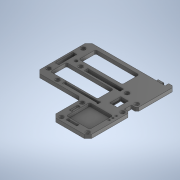
# Autodesk Inventor part: Cockpit_side_frame
Saved by Autodesk Inventor 2020.4 (Build 244396000, 396)
## iProperties
Created: 2022-01-27
Part Number: Cockpit_side_frame
Material: アセタール樹脂、黒
Document SubType Name: Modeling
Designer: Masato Kubotera
Density: 1.425 g/cm^3
Appearance: 滑らか - 黒
Mass: 53.6931 g
Surface Area: 240.102 cm^2
Volume: 37.6794 cm^3
Description: POM T5
Author: Masato Kubotera
Autodesk Inventor part; units mm, degrees
ref_plane "YZ Plane" through (0, 0, 0) normal (1, 0, 0) x (0, 1, 0)
ref_plane "XZ Plane" through (0, 0, 0) normal (0, 1, 0) x (-1, 0, 0)
ref_plane "XY Plane" through (0, 0, 0) normal (0, 0, 1) x (1, 0, 0)
derived "Trunk_basis.ipt"
sketch "スケッチ1" plane through (0, 0, 0) normal (0, 1, 0) x (-1, 0, 0)
  line L0 (0, 22) -> (0, -142.9) construction
  circle A0 centre (5, 0) radius 10.5 construction
  line L1 (-7, 16) -> (36, 16) construction
  line L2 (36, 16) -> (36, -16) construction
  line L3 (36, -16) -> (-7, -16) construction
  line L4 (-7, -16) -> (-7, 16) construction
  line L5 (-7, 16) -> (36, -16) construction
  line L6 (36, 16) -> (-7, -16) construction
  line L7 (33, 13.5) -> (6, 13.5) construction
  line L8 (6, 13.5) -> (6, -13.5) construction
  line L9 (6, -13.5) -> (33, -13.5) construction
  line L10 (33, -13.5) -> (33, 13.5) construction
  line L11 (33, 13.5) -> (6, -13.5) construction
  line L12 (6, 13.5) -> (33, -13.5) construction
  line L13 (-7, 0) -> (36, 0) construction
  arc A1 (5, 16) -> (-7, 10.583) centre (5, 0) ccw construction
  line L14 (34.5651, -16.05) -> (5, -16.05)
  line L15 (5, 16.05) -> (34.5651, 16.05)
  line L16 (36.05, 14.5651) -> (36.05, -14.5651)
  line L17 (36.05, -16.05) -> (-7.05, 16.05) construction
  line L18 (-7.05, -16.05) -> (36.05, 16.05) construction
  arc A2 (5, 16.05) -> (-6.5314, 11.1638) centre (5, 0) ccw
  arc A3 (-6.5314, 11.1638) -> (-7.05, 9.8372) centre (-6.0721, 10.2196) ccw
  arc A4 (36.05, 14.5651) -> (34.5651, 16.05) centre (35.3075, 15.3075) ccw
  circle A5 centre (6, 13.5) radius 1.35
  line L19 (19.5, 13.5) -> (19.5, -13.5) construction
  circle A6 centre (33, 13.5) radius 1.35
  line L20 (-15, 22) -> (-20, 17)
  line L21 (-20, 17) -> (-20, -19)
  line L22 (-20, -19) -> (-28.5, -27.5)
  line L23 (-28.5, -27.5) -> (-28.5, -103)
  line L24 (57.5, -22.5) -> (57.5, 17)
  line L25 (57.5, 17) -> (52.5, 22)
  line L26 (52.5, 22) -> (-15, 22)
  line L27 (-35.5597, -116.5529) -> (-28.5, -142.9)
  line L28 (-16, -139) -> (-16, -94) construction
  line L29 (-7.5, -140.4849) -> (-7.5, -142.9)
  line L30 (-7.5, -142.9) -> (7.5, -142.9)
  line L31 (7.5, -140.4849) -> (7.5, -142.9)
  arc A7 (-7.5, -140.4849) -> (-8.9849, -139) centre (-8.2425, -139.7425) ccw
  line L32 (-17.5, -138.9955) -> (-17.5, -133) construction
  line L33 (-19, -133) -> (-16, -133) construction
  line L34 (-19, -133) -> (-19, -139) construction
  line L35 (-16, -133) -> (-16, -139) construction
  line L36 (-15, 22) -> (-10, 22) construction
  line L37 (-10, 22) -> (-10, -22) construction
  line L38 (-10, -22) -> (-15, -22) construction
  line L39 (-15, -22) -> (-15, 22) construction
  line L40 (-15, 22) -> (-10, -22) construction
  line L41 (-10, 22) -> (-15, -22) construction
  line L42 (-12.5, 22) -> (-12.5, -22) construction
  line L43 (-10, 0) -> (-15, 0) construction
  circle A8 centre (-12.5, 17.75) radius 1.6
  line L44 (-15, 10) -> (-12.5, 10) construction
  line L45 (-12.5, 10) -> (-12.5, -10) construction
  line L46 (-12.5, -10) -> (-15, -10) construction
  line L47 (-15, -10) -> (-15, 10) construction
  line L48 (-15, 10) -> (-12.5, -10) construction
  line L49 (-12.5, 10) -> (-15, -10) construction
  line L50 (-12.45, 10.05) -> (-15.05, 10.05)
  line L51 (-15.05, 7.95) -> (-15.05, -7.95)
  line L52 (-15.05, -10.05) -> (-12.45, -10.05)
  line L53 (-12.45, -7.95) -> (-12.45, 7.95)
  line L54 (-12.45, 10.05) -> (-15.05, -10.05) construction
  line L55 (-15.05, 10.05) -> (-12.45, -10.05) construction
  arc A9 (-15.05, 10.05) -> (-15.05, 7.95) centre (-15.05, 9) ccw
  line L56 (-13.75, 10) -> (-13.75, -10) construction
  arc A10 (-12.45, 7.95) -> (-12.45, 10.05) centre (-12.45, 9) ccw
  circle A11 centre (-12.5, -17.75) radius 1.6
  arc A12 (-15.05, -7.95) -> (-15.05, -10.05) centre (-15.05, -9) ccw
  arc A13 (-12.45, -10.05) -> (-12.45, -7.95) centre (-12.45, -9) ccw
  line L57 (36, 14.4) -> (44.5, 14.4) construction
  line L58 (44.5, 14.4) -> (44.5, -14.4) construction
  line L59 (36, -14.4) -> (44.5, -14.4) construction
  line L60 (49.95, 7.95) -> (49.95, -7.95)
  line L61 (52.5, 0) -> (47.5, 0) construction
  line L62 (47.5, 22) -> (52.5, 22) construction
  line L63 (52.55, -7.95) -> (52.55, 7.95)
  line L64 (51.25, 10) -> (51.25, -10) construction
  line L65 (52.5, 10) -> (50, -10) construction
  line L66 (52.5, -10) -> (50, -10) construction
  line L67 (52.5, 10) -> (52.5, -10) construction
  line L68 (50, 10) -> (52.5, -10) construction
  line L69 (49.95, -10.05) -> (52.55, -10.05)
  line L70 (49.95, 10.05) -> (52.55, -10.05) construction
  line L71 (52.55, 10.05) -> (49.95, -10.05) construction
  line L72 (52.5, -22) -> (47.5, -22) construction
  line L73 (47.5, 22) -> (52.5, -22) construction
  line L74 (52.5, 22) -> (52.5, -22) construction
  line L75 (52.5, 22) -> (47.5, -22) construction
  line L76 (50, 22) -> (50, -22) construction
  line L77 (47.5, -22) -> (47.5, 22) construction
  circle A14 centre (50, -17.75) radius 1.6
  arc A15 (52.55, -10.05) -> (52.55, -7.95) centre (52.55, -9) ccw
  line L78 (50, -10) -> (50, 10) construction
  arc A16 (49.95, -7.95) -> (49.95, -10.05) centre (49.95, -9) ccw
  arc A17 (49.95, 10.05) -> (49.95, 7.95) centre (49.95, 9) ccw
  arc A18 (52.55, 7.95) -> (52.55, 10.05) centre (52.55, 9) ccw
  line L79 (50, 10) -> (52.5, 10) construction
  line L80 (52.55, 10.05) -> (49.95, 10.05)
  circle A19 centre (50, 17.75) radius 1.6
  circle A20 centre (5, 0) radius 16 construction
  arc A21 (-6.5314, -11.1638) -> (5, -16.05) centre (5, 0) ccw
  arc A22 (-7.05, -9.8372) -> (-6.5314, -11.1638) centre (-6.0721, -10.2196) ccw
  arc A23 (34.5651, -16.05) -> (36.05, -14.5651) centre (35.3075, -15.3075) ccw
  line L81 (-7.05, -9.8372) -> (-7.05, 9.8372)
  line L82 (17.5, -138.9955) -> (17.5, -133) construction
  line L83 (19, -133) -> (19, -139) construction
  line L84 (16, -133) -> (16, -139) construction
  line L85 (19, -133) -> (16, -133) construction
  circle A24 centre (6, -13.5) radius 1.35
  circle A25 centre (33, -13.5) radius 1.35
  line L86 (-25.5, -142.9) -> (-7.5, -142.9) construction
  line L87 (25.5, -142.9) -> (7.5, -142.9) construction
  line L88 (-23.5, -22.5) -> (57.5, -22.5) construction
  line L89 (57.5, -22.5) -> (57.5, -103)
  circle A26 centre (-13.5, -55) radius 1.75
  line L90 (-16.5, -59) -> (45.5, -59)
  line L91 (47.5, -61) -> (47.5, -88)
  line L92 (45.5, -90) -> (-16.5, -90)
  line L93 (-18.5, -88) -> (-18.5, -61)
  line L94 (-18.5, -59) -> (47.5, -90) construction
  line L95 (47.5, -59) -> (-18.5, -90) construction
  line L96 (-16.5, -27.5) -> (45.5, -27.5)
  line L97 (47.5, -29.5) -> (47.5, -49)
  line L98 (45.5, -51) -> (-16.5, -51)
  line L99 (-18.5, -49) -> (-18.5, -29.5)
  line L100 (-18.5, -27.5) -> (47.5, -51) construction
  line L101 (47.5, -27.5) -> (-18.5, -51) construction
  line L102 (-23.5, -108) -> (-28.5, -103)
  circle A27 centre (-20.5415, -102) radius 1.6
  line L103 (-25.7227, -96) -> (25.7227, -96)
  line L104 (25.7227, -96) -> (34.9603, -112)
  line L105 (35.5597, -116.5529) -> (28.5, -142.9)
  line L106 (-25.7227, -96) -> (-34.9603, -112)
  line L107 (57.5, -103) -> (52.5, -108)
  arc A28 (-16.5, -27.5) -> (-18.5, -29.5) centre (-16.5, -29.5) ccw
  arc A29 (-18.5, -49) -> (-16.5, -51) centre (-16.5, -49) ccw
  arc A30 (45.5, -51) -> (47.5, -49) centre (45.5, -49) ccw
  arc A31 (47.5, -29.5) -> (45.5, -27.5) centre (45.5, -29.5) ccw
  arc A32 (-16.5, -59) -> (-18.5, -61) centre (-16.5, -61) ccw
  arc A33 (-18.5, -88) -> (-16.5, -90) centre (-16.5, -88) ccw
  arc A34 (45.5, -90) -> (47.5, -88) centre (45.5, -88) ccw
  arc A35 (47.5, -61) -> (45.5, -59) centre (45.5, -61) ccw
  line L108 (-23.5, -108) -> (52.5, -108)
  line L109 (-25.5, -139) -> (-25.5, -142.9)
  line L110 (-25.5, -142.9) -> (-28.5, -142.9)
  line L111 (-17.9813, -99.3843) -> (-16.9961, -101.0907)
  line L112 (-16.9961, -102.9093) -> (-17.9813, -104.6157)
  line L113 (-19.5563, -105.525) -> (-21.5266, -105.525)
  line L114 (-23.1016, -104.6157) -> (-24.0868, -102.9093)
  line L115 (-24.0868, -101.0907) -> (-23.1016, -99.3843)
  line L116 (-21.5266, -98.475) -> (-19.5563, -98.475)
  line L117 (-16, -94) -> (16, -94) construction
  arc A36 (-24.0868, -101.0907) -> (-24.0868, -102.9093) centre (-23.5618, -102) ccw
  arc A37 (-23.1016, -104.6157) -> (-21.5266, -105.525) centre (-22.0516, -104.6157) ccw
  arc A38 (-19.5563, -105.525) -> (-17.9813, -104.6157) centre (-19.0313, -104.6157) ccw
  arc A39 (-16.9961, -102.9093) -> (-16.9961, -101.0907) centre (-17.5211, -102) ccw
  arc A40 (-17.9813, -99.3843) -> (-19.5563, -98.475) centre (-19.0313, -99.3843) ccw
  arc A41 (-21.5266, -98.475) -> (-23.1016, -99.3843) centre (-22.0516, -99.3843) ccw
  line L118 (16, -139) -> (16, -94) construction
  line L119 (16, -94) -> (-16, -94) construction
  line L120 (-25.5, -139) -> (-8.9849, -139)
  line L121 (25.5, -142.9) -> (28.5, -142.9)
  arc A42 (8.9849, -139) -> (7.5, -140.4849) centre (8.2425, -139.7425) ccw
  circle A43 centre (29.7641, -115) radius 1.25
  line L122 (33.4891, -124.2803) -> (21.898, -121.1745) construction
  line L123 (29.7641, -115) -> (25.623, -130.4548) construction
  circle A44 centre (29.7641, -115) radius 6 construction
  circle A45 centre (-20.5415, -102) radius 6 construction
  line L124 (1.9319, -109.4824) -> (7.5588, -130.4824)
  line L125 (5.6269, -133) -> (-5.6269, -133)
  line L126 (5.3151, -110.5176) -> (10.942, -131.5176)
  line L127 (12.8739, -133) -> (17.1947, -133)
  line L128 (19.1266, -131.5176) -> (24.7535, -110.5176)
  line L129 (22.8217, -108) -> (7.2469, -108)
  circle A46 centre (25.623, -130.4548) radius 1.25
  circle A47 centre (25.623, -130.4548) radius 6 construction
  line L130 (-1.9319, -109.4824) -> (-7.5588, -130.4824)
  arc A48 (1.9319, -109.4824) -> (-1.9319, -109.4824) centre (0, -110) ccw
  arc A49 (-7.5588, -130.4824) -> (-5.6269, -133) centre (-5.6269, -131) ccw
  arc A50 (5.6269, -133) -> (7.5588, -130.4824) centre (5.6269, -131) ccw
  arc A51 (7.2469, -108) -> (5.3151, -110.5176) centre (7.2469, -110) ccw
  arc A52 (24.7535, -110.5176) -> (22.8217, -108) centre (22.8217, -110) ccw
  arc A53 (17.1947, -133) -> (19.1266, -131.5176) centre (17.1947, -131) ccw
  arc A54 (10.942, -131.5176) -> (12.8739, -133) centre (12.8739, -131) ccw
  arc A55 (-5.3151, -110.5176) -> (-7.2469, -108) centre (-7.2469, -110) ccw
  line L131 (-22.8217, -108) -> (-7.2469, -108)
  line L132 (-5.3151, -110.5176) -> (-10.942, -131.5176)
  arc A56 (-22.8217, -108) -> (-24.7535, -110.5176) centre (-22.8217, -110) ccw
  line L133 (-19.1266, -131.5176) -> (-24.7535, -110.5176)
  arc A57 (-19.1266, -131.5176) -> (-17.1947, -133) centre (-17.1947, -131) ccw
  line L134 (-12.8739, -133) -> (-17.1947, -133)
  arc A58 (-12.8739, -133) -> (-10.942, -131.5176) centre (-12.8739, -131) ccw
  circle A59 centre (-29.7641, -115) radius 1.25
  circle A60 centre (-25.623, -130.4548) radius 1.25
  arc A61 (35.5597, -116.5529) -> (34.9603, -112) centre (29.7641, -115) ccw
  arc A62 (-34.9603, -112) -> (-35.5597, -116.5529) centre (-29.7641, -115) ccw
  arc A63 (-24.0151, -139) -> (-25.5, -140.4849) centre (-24.7575, -139.7425) ccw
  line L135 (25.5, -139) -> (25.5, -142.9)
  arc A64 (25.5, -140.4849) -> (24.0151, -139) centre (24.7575, -139.7425) ccw
  line L136 (25.5, -139) -> (8.9849, -139)
  line L137 (21.5266, -98.475) -> (19.5563, -98.475)
  line L138 (16.9961, -102.9093) -> (17.9813, -104.6157)
  arc A65 (21.5266, -105.525) -> (23.1016, -104.6157) centre (22.0516, -104.6157) ccw
  circle A66 centre (20.5415, -102) radius 1.6
  line L139 (24.0868, -101.0907) -> (23.1016, -99.3843)
  arc A67 (24.0868, -102.9093) -> (24.0868, -101.0907) centre (23.5618, -102) ccw
  line L140 (23.1016, -104.6157) -> (24.0868, -102.9093)
  arc A68 (23.1016, -99.3843) -> (21.5266, -98.475) centre (22.0516, -99.3843) ccw
  line L141 (19.5563, -105.525) -> (21.5266, -105.525)
  arc A69 (19.5563, -98.475) -> (17.9813, -99.3843) centre (19.0313, -99.3843) ccw
  arc A70 (17.9813, -104.6157) -> (19.5563, -105.525) centre (19.0313, -104.6157) ccw
  line L142 (17.9813, -99.3843) -> (16.9961, -101.0907)
  arc A71 (16.9961, -101.0907) -> (16.9961, -102.9093) centre (17.5211, -102) ccw
  line L143 (16, -139) -> (16, -94) construction
  circle A72 centre (20.5415, -102) radius 6 construction
  arc A73 (29.5045, -117.5445) -> (31.2612, -117.0738) centre (30.247, -116.802) ccw construction
  line L144 (31.8379, -116.4971) -> (31.2612, -117.0738) construction
  line L145 (29.5045, -117.5445) -> (28.7167, -117.3334) construction
  arc A74 (27.4307, -116.0474) -> (28.7167, -117.3334) centre (28.4449, -116.3192) ccw construction
  line L146 (27.4307, -116.0474) -> (27.2196, -115.2596) construction
  line L147 (27.6903, -113.5029) -> (28.267, -112.9262) construction
  arc A75 (30.0237, -112.4555) -> (28.267, -112.9262) centre (29.2813, -113.198) ccw construction
  arc A76 (27.6903, -113.5029) -> (27.2196, -115.2596) centre (27.9621, -114.5171) ccw construction
  line L148 (30.0237, -112.4555) -> (30.8116, -112.6666) construction
  arc A77 (31.8379, -116.4971) -> (32.3086, -114.7404) centre (31.5662, -115.4829) ccw construction
  arc A78 (32.0975, -113.9526) -> (30.8116, -112.6666) centre (31.0833, -113.6808) ccw construction
  line L149 (32.0975, -113.9526) -> (32.3086, -114.7404) construction
  line L150 (-20.5415, -102) -> (20.5415, -102) construction
  circle A79 centre (0, -102) radius 1.6
  line L151 (0.4078, -104.525) -> (-0.4078, -104.525)
  arc A80 (-0.4078, -99.475) -> (-1.9828, -100.3843) centre (-0.9328, -100.3843) ccw
  arc A81 (0.4078, -104.525) -> (1.9828, -103.6157) centre (0.9328, -103.6157) ccw
  line L152 (2.3906, -102.9093) -> (1.9828, -103.6157)
  line L153 (-0.4078, -99.475) -> (0.4078, -99.475)
  arc A82 (1.9828, -100.3843) -> (0.4078, -99.475) centre (0.9328, -100.3843) ccw
  line L154 (1.9828, -100.3843) -> (2.3906, -101.0907)
  arc A83 (2.3906, -102.9093) -> (2.3906, -101.0907) centre (1.8656, -102) ccw
  line L155 (-2.3906, -101.0907) -> (-1.9828, -100.3843)
  arc A84 (-2.3906, -101.0907) -> (-2.3906, -102.9093) centre (-1.8656, -102) ccw
  line L156 (-1.9828, -103.6157) -> (-2.3906, -102.9093)
  arc A85 (-1.9828, -103.6157) -> (-0.4078, -104.525) centre (-0.9328, -103.6157) ccw
  circle A86 centre (0, -102) radius 1.25
  point P0 (0, 0)
  point P1 (14.5, 0)
  point P2 (19.5, 0)
  point P3 (-7.05, 10.6019)
  point P4 (19.5, 0)
  point P5 (-12.5, 0)
  point P6 (-13.75, 0)
  point P7 (36.05, 14.4)
  point P8 (36.05, -14.4)
  point P9 (51.25, 0)
  point P10 (50, 0)
  point P11 (14.5, -74.5)
  point P12 (14.5, -39.25)
  point P13 (-18.5063, -98.475)
  point P14 (-16.4711, -102)
  point P15 (-18.5063, -105.525)
  point P16 (-22.5766, -105.525)
  point P17 (-22.5766, -98.475)
  point P18 (-24.6118, -102)
  point P19 (-22.5766, -105.525)
  point P20 (-18.5063, -105.525)
  point P21 (-16.4711, -102)
  point P22 (-18.5063, -98.475)
  point P23 (-22.5766, -98.475)
  point P24 (27.6936, -122.7274)
  point P25 (0, -102.2726)
  point P26 (0, -133)
  point P27 (-7.5, -139)
  point P28 (-22.5766, -98.475)
  point P29 (18.5063, -98.475)
  point P30 (18.5063, -98.475)
  point P31 (22.5766, -105.525)
  point P32 (22.5766, -105.525)
  point P33 (24.6118, -102)
  point P34 (22.5766, -98.475)
  point P35 (22.5766, -98.475)
  point P36 (22.5766, -98.475)
  point P37 (18.5063, -105.525)
  point P38 (16.4711, -102)
  point P39 (16.4711, -102)
  point P40 (18.5063, -105.525)
  point P41 (29.7641, -115)
  point P42 (29.7641, -115)
  point P43 (30.5187, -117.8163)
  point P44 (30.5187, -117.8163)
  point P45 (27.7025, -117.0617)
  point P46 (27.7025, -117.0617)
  point P47 (31.8258, -112.9383)
  point P48 (26.9479, -114.2454)
  point P49 (29.0095, -112.1837)
  point P50 (29.0095, -112.1837)
  point P51 (31.8258, -112.9383)
  point P52 (29.0095, -112.1837)
  point P53 (32.5804, -115.7546)
  point P54 (-1.4578, -99.475)
  point P55 (-1.4578, -99.475)
  point P56 (-1.4578, -99.475)
  point P57 (1.4578, -104.525)
  point P58 (1.4578, -99.475)
  point P59 (1.4578, -99.475)
  point P60 (2.9156, -102)
  point P61 (-2.9156, -102)
  point P62 (-1.4578, -104.525)
  point P63 (-1.4578, -104.525)
sketch "スケッチ2" plane through (0, 0, 0) normal (0, 1, 0) x (-1, 0, 0)
  line L0 (-28.5, -22.5) -> (86.5, -22.5) construction
  line L1 (86.5, -22.5) -> (86.5, -138.5)
  line L2 (86.5, -96) -> (-28.5, -96) construction
  line L3 (-28.5, -96) -> (-28.5, -22.5) construction
  line L4 (-28.5, -22.5) -> (86.5, -96) construction
  line L5 (86.5, -22.5) -> (-28.5, -96) construction
  line L6 (36.5, -101) -> (36.5, -133.5)
  line L7 (41.5, -138.5) -> (86.5, -138.5)
  line L8 (61.9, -67.85) -> (71.1, -67.85) construction
  line L9 (71.1, -67.85) -> (71.1, -81.65) construction
  line L10 (71.1, -81.65) -> (61.9, -81.65) construction
  line L11 (61.9, -81.65) -> (61.9, -67.85) construction
  line L12 (61.9, -67.85) -> (71.1, -81.65) construction
  line L13 (71.1, -67.85) -> (61.9, -81.65) construction
  line L14 (61.2, -67.2) -> (71.8, -67.2) construction
  line L15 (71.8, -67.2) -> (71.8, -82.3) construction
  line L16 (71.8, -82.3) -> (61.2, -82.3) construction
  line L17 (61.2, -82.3) -> (61.2, -67.2) construction
  line L18 (61.2, -67.2) -> (71.8, -82.3) construction
  line L19 (71.8, -67.2) -> (61.2, -82.3) construction
  line L20 (66.5, -67.2) -> (66.5, -82.3) construction
  line L21 (71.8, -74.75) -> (61.2, -74.75) construction
  line L22 (62.6349, -67.15) -> (70.3651, -67.15)
  line L23 (61.15, -68.6349) -> (61.15, -80.8651)
  line L24 (63.3349, -67.8) -> (69.6651, -67.8)
  line L25 (61.85, -69.2849) -> (61.85, -80.2151)
  arc A0 (62.6349, -67.15) -> (61.15, -68.6349) centre (61.8925, -67.8925) ccw
  arc A1 (63.3349, -67.8) -> (61.85, -69.2849) centre (62.5925, -68.5425) ccw
  arc A2 (71.85, -68.6349) -> (70.3651, -67.15) centre (71.1075, -67.8925) ccw
  arc A3 (71.15, -69.2849) -> (69.6651, -67.8) centre (70.4075, -68.5425) ccw
  line L26 (62.6349, -82.35) -> (70.3651, -82.35)
  line L27 (63.3349, -81.7) -> (69.6651, -81.7)
  arc A4 (61.85, -80.2151) -> (63.3349, -81.7) centre (62.5925, -80.9575) ccw
  arc A5 (61.15, -80.8651) -> (62.6349, -82.35) centre (61.8925, -81.6075) ccw
  arc A6 (70.3651, -82.35) -> (71.85, -80.8651) centre (71.1075, -81.6075) ccw
  arc A7 (69.6651, -81.7) -> (71.15, -80.2151) centre (70.4075, -80.9575) ccw
  line L28 (71.15, -69.2849) -> (71.15, -80.2151)
  line L29 (71.85, -68.6349) -> (71.85, -80.8651)
  line L30 (-23.5, -22.5) -> (-28.5, -27.5)
  line L31 (-28.5, -59.25) -> (86.5, -59.25) construction
  line L32 (29, -22.5) -> (29, -96) construction
  line L33 (-23.5, -96) -> (-28.5, -91)
  line L34 (-28.5, -27.5) -> (-28.5, -91)
  line L35 (-21, -25) -> (-26, -25) construction
  line L36 (-26, -25) -> (-26, -93.5) construction
  line L37 (-26, -93.5) -> (-21, -93.5) construction
  line L38 (-21, -93.5) -> (-21, -25) construction
  line L39 (-21, -25) -> (-26, -93.5) construction
  line L40 (-26, -25) -> (-21, -93.5) construction
  line L41 (-26.05, -46.7) -> (-20.95, -46.7)
  line L42 (-20.95, -46.7) -> (-20.95, -71.8)
  line L43 (-20.95, -71.8) -> (-26.05, -71.8)
  line L44 (-26.05, -71.8) -> (-26.05, -46.7)
  line L45 (-26.05, -46.7) -> (-20.95, -71.8) construction
  line L46 (-20.95, -46.7) -> (-26.05, -71.8) construction
  line L47 (-26, -46.75) -> (-21, -46.75) construction
  line L48 (-26, -71.75) -> (-21, -71.75) construction
  line L49 (-23.5, -25) -> (-23.5, -93.5) construction
  circle A8 centre (-23.5, -35) radius 3
  circle A9 centre (-23.5, -35) radius 1.6
  arc A10 (-24.5651, -46.7) -> (-26.05, -48.1849) centre (-25.3075, -47.4425) ccw
  arc A11 (-20.95, -48.1849) -> (-22.4349, -46.7) centre (-21.6925, -47.4425) ccw
  arc A12 (-26.05, -70.3151) -> (-24.5651, -71.8) centre (-25.3075, -71.0575) ccw
  arc A13 (-22.4349, -71.8) -> (-20.95, -70.3151) centre (-21.6925, -71.0575) ccw
  circle A14 centre (-23.5, -83.5) radius 3
  circle A15 centre (-23.5, -83.5) radius 1.6
  line L50 (31.5, -96) -> (36.5, -101)
  line L51 (-23.5, -96) -> (31.5, -96)
  line L52 (79, -61) -> (-21, -61) construction
  line L53 (-21, -61) -> (-21, -56) construction
  line L54 (-21, -56) -> (79, -56) construction
  line L55 (79, -56) -> (79, -61) construction
  line L56 (79, -61) -> (-21, -56) construction
  line L57 (-21, -61) -> (79, -56) construction
  line L58 (-21, -58.5) -> (79, -58.5) construction
  line L59 (29, -56) -> (29, -61) construction
  line L60 (4, -56) -> (4, -61) construction
  line L61 (54.05, -55.95) -> (3.95, -55.95)
  line L62 (3.95, -55.95) -> (3.95, -61.05)
  line L63 (3.95, -61.05) -> (54.05, -61.05)
  line L64 (54.05, -61.05) -> (54.05, -55.95)
  line L65 (54.05, -55.95) -> (3.95, -61.05) construction
  line L66 (3.95, -55.95) -> (54.05, -61.05) construction
  arc A16 (5.4349, -55.95) -> (3.95, -57.4349) centre (4.6925, -56.6925) ccw
  circle A17 centre (-3.5, -58.5) radius 3
  circle A18 centre (-3.5, -58.5) radius 1.6
  line L67 (54, -56) -> (54, -61) construction
  arc A19 (54.05, -57.4349) -> (52.5651, -55.95) centre (53.3075, -56.6925) ccw
  circle A20 centre (61.5, -58.5) radius 3
  circle A21 centre (61.5, -58.5) radius 1.6
  arc A22 (3.95, -59.5651) -> (5.4349, -61.05) centre (4.6925, -60.3075) ccw
  arc A23 (52.5651, -61.05) -> (54.05, -59.5651) centre (53.3075, -60.3075) ccw
  line L68 (-21, -88.5) -> (79, -88.5) construction
  line L69 (79, -88.5) -> (79, -93.5) construction
  line L70 (79, -93.5) -> (-21, -93.5) construction
  line L71 (-21, -93.5) -> (-21, -88.5) construction
  line L72 (-21, -88.5) -> (79, -93.5) construction
  line L73 (79, -88.5) -> (-21, -93.5) construction
  line L74 (-21, -91) -> (79, -91) construction
  line L75 (29, -88.5) -> (29, -93.5) construction
  line L76 (54.05, -91.05) -> (3.95, -91.05)
  line L77 (3.95, -91.05) -> (3.95, -88.45)
  line L78 (3.95, -88.45) -> (54.05, -88.45)
  line L79 (54.05, -88.45) -> (54.05, -91.05)
  line L80 (54.05, -91.05) -> (3.95, -88.45) construction
  line L81 (3.95, -91.05) -> (54.05, -88.45) construction
  line L82 (4, -88.5) -> (4, -91) construction
  line L83 (54, -88.5) -> (54, -91) construction
  line L84 (4, -89.75) -> (54, -89.75) construction
  arc A24 (6.05, -88.45) -> (3.95, -88.45) centre (5, -88.45) ccw
  arc A25 (54.05, -88.45) -> (51.95, -88.45) centre (53, -88.45) ccw
  arc A26 (3.95, -91.05) -> (6.05, -91.05) centre (5, -91.05) ccw
  arc A27 (51.95, -91.05) -> (54.05, -91.05) centre (53, -91.05) ccw
  circle A28 centre (-3.5, -91) radius 3
  circle A29 centre (-3.5, -91) radius 1.6
  circle A30 centre (61.5, -91) radius 3 construction
  circle A31 centre (61.5, -91) radius 1.6 construction
  line L85 (-23.5, -22.5) -> (64.25, -22.5)
  line L86 (64.25, -22.5) -> (64.25, -17.5)
  line L87 (64.25, -17.5) -> (72.25, -17.5)
  line L88 (72.25, -17.5) -> (72.25, -22.5)
  line L89 (72.25, -22.5) -> (79, -22.5)
  line L90 (79, -22.5) -> (79, -17.5)
  line L91 (86.5, -22.5) -> (86.5, -20)
  line L92 (79, -17.5) -> (84, -17.5)
  line L93 (84, -17.5) -> (86.5, -20)
  line L94 (68.25, -17.5) -> (68.25, -22.5) construction
  arc A32 (62.7651, -22.5) -> (64.25, -21.0151) centre (63.5075, -21.7575) ccw
  arc A33 (72.25, -21.0151) -> (73.7349, -22.5) centre (72.9925, -21.7575) ccw
  arc A34 (77.5151, -22.5) -> (79, -21.0151) centre (78.2575, -21.7575) ccw
  line L95 (-16, -88.5) -> (-16, -68.5) construction
  line L96 (-16, -68.5) -> (64, -68.5) construction
  line L97 (64, -68.5) -> (64, -88.5) construction
  line L98 (45.5, -86) -> (-16.5, -86)
  line L99 (-18.5, -84) -> (-18.5, -65.5)
  line L100 (-16.5, -63.5) -> (45.5, -63.5)
  line L101 (47.5, -65.5) -> (47.5, -84)
  line L102 (47.5, -86) -> (-18.5, -63.5) construction
  line L103 (-18.5, -86) -> (47.5, -63.5) construction
  arc A35 (-16.5, -63.5) -> (-18.5, -65.5) centre (-16.5, -65.5) ccw
  arc A36 (-18.5, -84) -> (-16.5, -86) centre (-16.5, -84) ccw
  arc A37 (45.5, -86) -> (47.5, -84) centre (45.5, -84) ccw
  arc A38 (47.5, -65.5) -> (45.5, -63.5) centre (45.5, -65.5) ccw
  line L104 (36.5, -133.5) -> (41.5, -138.5)
  line L105 (44, -131) -> (39, -131) construction
  line L106 (39, -131) -> (39, -96) construction
  line L107 (39, -96) -> (44, -96) construction
  line L108 (44, -96) -> (44, -131) construction
  line L109 (44, -131) -> (39, -96) construction
  line L110 (39, -131) -> (44, -96) construction
  line L111 (41.5, -96) -> (41.5, -131) construction
  line L112 (39, -113.5) -> (44, -113.5) construction
  line L113 (41.5, -107.5) -> (44, -107.5) construction
  line L114 (41.45, -107.45) -> (44.05, -107.45)
  line L115 (44.05, -107.45) -> (44.05, -119.55)
  line L116 (44.05, -119.55) -> (41.45, -119.55)
  line L117 (41.45, -119.55) -> (41.45, -107.45)
  line L118 (41.45, -107.45) -> (44.05, -119.55) construction
  line L119 (44.05, -107.45) -> (41.45, -119.55) construction
  arc A39 (44.05, -109.55) -> (44.05, -107.45) centre (44.05, -108.5) ccw
  arc A40 (42.9349, -107.45) -> (41.45, -108.9349) centre (42.1925, -108.1925) ccw
  line L120 (41.5, -119.5) -> (44, -119.5) construction
  arc A41 (44.05, -119.55) -> (44.05, -117.45) centre (44.05, -118.5) ccw
  arc A42 (41.45, -118.0651) -> (42.9349, -119.55) centre (42.1925, -118.8075) ccw
  line L121 (42.75, -107.5) -> (42.75, -119.5) construction
  circle A43 centre (41.5, -125.5) radius 3 construction
  circle A44 centre (41.5, -125.5) radius 1.6 construction
  circle A45 centre (41.5, -101.5) radius 3
  circle A46 centre (41.5, -101.5) radius 1.6
  circle A47 centre (-13.5, -55) radius 2
  line L122 (39, -131) -> (77.8645, -131) construction
  line L123 (77.8645, -131) -> (77.8645, -136) construction
  line L124 (77.8645, -136) -> (39, -136) construction
  line L125 (39, -136) -> (39, -131) construction
  line L126 (39, -131) -> (77.8645, -136) construction
  line L127 (77.8645, -131) -> (39, -136) construction
  line L128 (39, -133.5) -> (77.8645, -133.5) construction
  line L129 (58.4322, -131) -> (58.4322, -136) construction
  line L130 (58.4322, -133.5) -> (58.4322, -131) construction
  line L131 (50.8822, -130.95) -> (65.9822, -130.95)
  line L132 (65.9822, -130.95) -> (65.9822, -133.55)
  line L133 (65.9822, -133.55) -> (50.8822, -133.55)
  line L134 (50.8822, -133.55) -> (50.8822, -130.95)
  line L135 (50.8822, -130.95) -> (65.9822, -133.55) construction
  line L136 (65.9822, -130.95) -> (50.8822, -133.55) construction
  line L137 (50.9322, -131) -> (50.9322, -133.5) construction
  arc A48 (52.9822, -130.95) -> (50.8822, -130.95) centre (51.9322, -130.95) ccw
  arc A49 (50.8822, -132.0651) -> (52.3672, -133.55) centre (51.6247, -132.8075) ccw
  arc A50 (65.9822, -130.95) -> (63.8822, -130.95) centre (64.9322, -130.95) ccw
  arc A51 (64.4973, -133.55) -> (65.9822, -132.0651) centre (65.2398, -132.8075) ccw
  line L138 (65.9322, -131) -> (65.9322, -133.5) construction
  line L139 (50.9322, -132.25) -> (65.9322, -132.25) construction
  circle A52 centre (72.4322, -133.5) radius 1.6 construction
  circle A53 centre (72.4322, -133.5) radius 3 construction
  circle A54 centre (44.4322, -133.5) radius 1.6
  circle A55 centre (44.4322, -133.5) radius 3
  line L140 (48.5, -96) -> (77, -96)
  line L141 (79, -98) -> (79, -126.5)
  line L142 (77, -128.5) -> (48.5, -128.5)
  line L143 (46.5, -126.5) -> (46.5, -98)
  line L144 (46.5, -96) -> (79, -128.5) construction
  line L145 (79, -96) -> (46.5, -128.5) construction
  arc A56 (48.5, -96) -> (46.5, -98) centre (48.5, -98) ccw
  arc A57 (46.5, -126.5) -> (48.5, -128.5) centre (48.5, -126.5) ccw
  arc A58 (77, -128.5) -> (79, -126.5) centre (77, -126.5) ccw
  arc A59 (79, -98) -> (77, -96) centre (77, -98) ccw
  line L146 (79, -91.1738) -> (84, -91.1738) construction
  line L147 (84, -91.1738) -> (84, -136) construction
  line L148 (84, -136) -> (79, -136) construction
  line L149 (79, -136) -> (79, -91.1738) construction
  line L150 (79, -91.1738) -> (84, -136) construction
  line L151 (84, -91.1738) -> (79, -136) construction
  line L152 (81.5, -91.1738) -> (81.5, -136) construction
  circle A60 centre (81.5, -93.6738) radius 1.475
  circle A61 centre (81.5, -98.6738) radius 1.475
  circle A62 centre (81.5, -103.6738) radius 1.475
  circle A63 centre (81.5, -133.5) radius 1.6
  arc A64 (84, -91.1738) -> (79, -91.1738) centre (81.5, -133.5) ccw construction
  arc A65 (84.0111, -91.0742) -> (78.9889, -91.0742) centre (81.5, -133.5) ccw construction
  line L153 (86.5, -133.5) -> (81.5, -138.5)
  arc A66 (79, -131) -> (84, -136) centre (81.5, -133.5) ccw construction
  line L154 (79, -58.5) -> (84, -58.5) construction
  line L155 (84, -58.5) -> (84, -91) construction
  line L156 (84, -91) -> (79, -91) construction
  line L157 (79, -91) -> (79, -58.5) construction
  line L158 (79, -58.5) -> (84, -91) construction
  line L159 (84, -58.5) -> (79, -91) construction
  line L160 (79, -74.75) -> (84, -74.75) construction
  line L161 (81.5, -58.5) -> (81.5, -91) construction
  line L162 (79, -69.75) -> (84, -69.75) construction
  line L163 (78.95, -69.7) -> (86.5, -69.7)
  line L164 (84.05, -69.7) -> (84.05, -79.8) construction
  line L165 (84.05, -79.8) -> (78.95, -79.8)
  line L166 (78.95, -79.8) -> (78.95, -69.7)
  line L167 (78.95, -69.7) -> (84.05, -79.8) construction
  line L168 (84.05, -69.7) -> (78.95, -79.8) construction
  arc A67 (80.4349, -69.7) -> (78.95, -71.1849) centre (79.6925, -70.4425) ccw
  arc A68 (78.95, -78.3151) -> (80.4349, -79.8) centre (79.6925, -79.0575) ccw
  line L169 (79, -79.75) -> (84, -79.75) construction
  circle A69 centre (81.5, -64.75) radius 1.6
  circle A70 centre (81.5, -64.75) radius 3
  circle A71 centre (81.5, -84.75) radius 1.6
  circle A72 centre (81.5, -84.75) radius 3
  line L170 (84.05, -79.8) -> (86.5, -79.8)
  circle A73 centre (81.5, -133.5) radius 3
  line L171 (75.625, -22.5) -> (75.625, -27.147) construction
  line L172 (60.875, -22.5) -> (60.875, -27.147) construction
  line L173 (64.25, -22.5) -> (72.25, -22.5)
  line L174 (-13.5, -29.5) -> (-13.5, -49)
  line L175 (-11.5, -51) -> (45.5, -51)
  line L176 (47.5, -49) -> (47.5, -29.5)
  line L177 (45.5, -27.5) -> (-11.5, -27.5)
  arc A74 (-11.5, -27.5) -> (-13.5, -29.5) centre (-11.5, -29.5) ccw
  arc A75 (-13.5, -49) -> (-11.5, -51) centre (-11.5, -49) ccw
  arc A76 (45.5, -51) -> (47.5, -49) centre (45.5, -49) ccw
  arc A77 (47.5, -29.5) -> (45.5, -27.5) centre (45.5, -29.5) ccw
  point P0 (0, 0)
  point P1 (29, -59.25)
  point P2 (-25.7227, -96)
  point P3 (66.5, -74.75)
  point P4 (61.15, -67.15)
  point P5 (61.85, -67.8)
  point P6 (-23.5, -59.25)
  point P7 (29, -58.5)
  point P8 (29, -91)
  point P9 (29, -89.75)
  point P10 (29, -89.75)
  point P11 (52.5, -22)
  point P12 (14.5, -74.75)
  point P13 (-18.5, -61)
  point P14 (47.5, -61)
  point P15 (41.5, -113.5)
  point P16 (42.75, -113.5)
  point P17 (58.4322, -133.5)
  point P18 (58.4322, -132.25)
  point P19 (73.7349, -22.5)
  point P20 (72.25, -21.0151)
  point P21 (64.4973, -133.55)
  point P22 (65.9822, -132.0651)
  point P23 (41.45, -118.0651)
  point P24 (-22.4349, -46.7)
  point P25 (-20.95, -70.3151)
  point P26 (-24.5651, -71.8)
  point P27 (54.05, -59.5651)
  point P28 (52.5651, -61.05)
  point P29 (5.4349, -61.05)
  point P30 (3.95, -59.5651)
  point P31 (52.5651, -55.95)
  point P32 (54.05, -57.4349)
  point P33 (51.95, -88.45)
  point P34 (51.95, -91.05)
  point P35 (6.05, -91.05)
  point P36 (62.75, -112.25)
  point P37 (81.5, -113.5869)
  point P38 (81.5, -74.75)
  point P39 (80.4349, -79.8)
  point P40 (78.95, -78.3151)
  point P41 (72.25, -22.5)
  point P42 (-13.5, -51)
  point P43 (47.5, -27.5)
  point P44 (-13.5, -27.5)
  dimension "d1" = 73.5
  dimension "d2" = 115
  dimension "d3" = 42.5
  dimension "d5" = 9.2
  dimension "d6" = 13.8
  dimension "d7" = 10.6
  dimension "d8" = 15.1
  dimension "d9" = 1.05
  dimension "d10" = 0.05
  dimension "d11" = 0.05
  dimension "d12" = 0.05
  dimension "d13" = 0.05
  dimension "d14" = 1.05
  dimension "d15" = 5
  dimension "d16" = 2.5
  dimension "d18" = 6
  dimension "d19" = 3.2
  dimension "d20" = 1.05
  dimension "d21" = 0.05
  dimension "d22" = 0.05
  dimension "d23" = 48.5
  dimension "d24" = 5
  dimension "d25" = 5
  dimension "d26" = 100
  dimension "d27" = 33.5
  dimension "d28" = 5
  dimension "d30" = 1.05
  dimension "d31" = 6
  dimension "d32" = 3.2
  dimension "d33" = 0.05
  dimension "d34" = 0.05
  dimension "d36" = 65
  dimension "d38" = 0.05
  dimension "d39" = 0.05
  dimension "d41" = 5
  dimension "d42" = 1.05
  dimension "d44" = 6
  dimension "d45" = 3.2
  dimension "d46" = 65
  dimension "d47" = 2.5
  dimension "d48" = 5
  dimension "d49" = 31.5
  dimension "d50" = 8
  dimension "d51" = 15.75
  dimension "d52" = 7.5
  dimension "d53" = 1.05
  dimension "d54" = 1.05
  dimension "d57" = 80
  dimension "d58" = 5
  dimension "d59" = 20
  dimension "d60" = 27.5
  dimension "d61" = 13.75
  dimension "d62" = 7.5
  dimension "d63" = 2.5
  dimension "d64" = 2.5
  dimension "d65" = 2
  dimension "d67" = 5
  dimension "d69" = 5
  dimension "d70" = 1.05
  dimension "d71" = 1.05
  dimension "d72" = 12
  dimension "d73" = 0.05
  dimension "d74" = 0.05
  dimension "d75" = 6
  constraints: 356 end point, 105 point on circle, 95 point on line, 86 symmetric about line, 81 midpoint, 78 centre point, 45 parallel, 35 perpendicular, 25 tangent, 19 horizontal, 16 coincident, 12 collinear, 9 equal radius, 9 vertical, 1 concentric, 39 other
  measures "d1" distance of L2.end L0.start
  measures "d2" distance of L0.start L0.end
  measures "d3" distance of L1.end L2.start
  measures "d5" distance of L9.end L11.start
  measures "d6" distance of L8.end L9.end
  measures "d7" distance of L15.end L19.end
  measures "d8" distance of L14.end L15.end
  measures "d9" radius of A0
  measures "d10" distance between parallel lines of L14 L22
  measures "d11" distance between parallel lines of L23 L17
  measures "d12" distance between parallel lines of L8 L24
  measures "d13" distance between parallel lines of L25 L11
  measures "d14" radius of A1
  measures "d15" distance of L35.start L35.end
  measures "d16" horizontal distance of L35.end L0.start
  measures "d18" diameter of A8
  measures "d19" diameter of A9
  measures "d20" radius of A10
  measures "d21" horizontal distance of L41.start L47.start
  measures "d22" horizontal distance of L47.start L41.start
  measures "d23" distance of A15.centre A8.centre
  measures "d24" horizontal distance of L33.start L33.end
  measures "d25" horizontal distance of L6.start L50.start
  measures "d26" distance of L53.end L54.end
  measures "d27" vertical distance of L0.end L54.end
  measures "d28" distance of L54.end L52.start
  measures "d30" radius of A16
  measures "d31" diameter of A17
  measures "d32" diameter of A18
  measures "d33" horizontal distance of L61.end L60.start
  measures "d34" horizontal distance of L60.start L61.end
  measures "d36" distance of A20.centre A18.centre
  measures "d38" horizontal distance of L77.end L82.start
  measures "d39" horizontal distance of L77.end L82.start
  measures "d41" distance of L68.end L69.end
  measures "d42" radius of A24
  measures "d44" diameter of A28
  measures "d45" diameter of A29
  measures "d46" distance of A30.centre A29.centre
  measures "d47" vertical distance of L91.end L90.end
  measures "d48" vertical distance of L0.end L90.end
  measures "d49" horizontal distance of point (52.5, -22) L92.end
  measures "d50" distance of L86.end L87.end
  measures "d51" horizontal distance of L92.end L94.end
  measures "d52" horizontal distance of L90.end L0.end
  measures "d53" radius of A32
  measures "d54" radius of A34
  measures "d57" distance of L95.end L96.end
  measures "d58" horizontal distance of L68.start L95.end
  measures "d59" distance of L96.end L97.end
  measures "d60" distance of L68.end L52.start
  measures "d61" vertical distance of point (66.5, -74.75) L52.start
  measures "d62" horizontal distance of L2.start L69.end
  measures "d63" distance from line of L102.end L52
  measures "d64" distance between parallel lines of L68 L98
  measures "d65" radius of A35
  measures "d67" horizontal distance of L7.start L6.end
  measures "d69" distance of L105.end L105.start
  measures "d70" radius of A40
  measures "d71" radius of A39
  measures "d72" distance of L120.end L113.end
  measures "d73" horizontal distance of L114.end L113.end
  measures "d74" horizontal distance of L114.end L113.end
  measures "d75" diameter of A43
extrude "押し出し1" add sketch "スケッチ2" along normal blind 5 contours L1 L163 A67 L166 A68 L165 L170 L153 L7 L104 L6 L50 L51 L33 L34 L30 L85 A32 L173 A33 L89 A34 L90 L92 L93 L91
extrude "押し出し2" add sketch "スケッチ2" along normal blind 3 contours A8 | A14 | A17 | A20 | A28 | A45 | A55 | A70 | A72 | A73
extrude "押し出し3" add sketch "スケッチ2" along normal blind 1.5 contours L22 A2 L29 A6 L26 A5 L23 A0
extrude "押し出し4" add sketch "スケッチ2" along normal blind 0.5 contours L140 A59 L141 A58 L142 A57 L143 A56
chamfer "面取り1" distance 2.5 angle 45 2 edges at (-86.5, 2.5, -79.8) (-86.5, 2.5, -69.7)
sketch "スケッチ3" plane through (-77.5151, 0, -22.5) normal (0, 0, 1) x (1, 0, 0)
  line L0 (-6.4849, 0) -> (-6.4849, 5) projected
  line L1 (1.8901, 0) -> (1.8901, 5)
  line L2 (0, 5) -> (3.7802, 5) projected
  line L3 (16.6401, 0) -> (16.6401, 5)
  line L4 (14.75, 5) -> (101.0151, 5) projected
  point P0 (77.5151, 0)
  point P1 (1.8901, 2.5)
  point P2 (16.6401, 2.5)
  point P3 (1.8901, 2.5)
  point P4 (16.6401, 2.5)
  constraints: 4 end point, 3 midpoint, 2 coincident, 1 parallel, 1 point on line
hole "穴1" at (-75.625, 2.5, -22.5) at (-60.875, 2.5, -22.5) direction (0, 0, -1) diameter 3.242 depth 5 tip angle 118 thread size "M4x0.7" class "6H" standard "ISO Metric profile"
extrude "押し出し5" add sketch "スケッチ2" along normal blind 2.5 contours L173 A32 L86 L87 L88 A33
equation "\"d11\" = d10"
equation "\"d12\" = d10"
equation "\"d13\" = d12"
equation "\"d14\" = d9"
equation "\"d22\" = d21"
equation "\"d25\" = d24"
equation "\"d30\" = d20"
equation "\"d31\" = d18"
equation "\"d32\" = d19"
equation "\"d33\" = d21"
equation "\"d34\" = d33"
equation "\"d38\" = d21"
equation "\"d39\" = d38"
equation "\"d41\" = d28"
